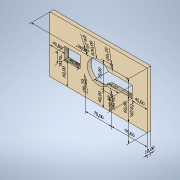
# Autodesk Inventor part: MotorHalterung
Saved by Autodesk Inventor 2020.3 (Build 243373010, 373A)
## iProperties
Created: 2021-02-04
Part Number: MotorHalterung
Material: Generisch
Document SubType Name: Modeling
Designer: Stefan
Density: 1 g/cm^3
Appearance: Vorgabe
Author: Stefan
Autodesk Inventor part; units mm, degrees
ref_plane "YZ Plane" through (0, 0, 0) normal (1, 0, 0) x (0, 1, 0)
ref_plane "XZ Plane" through (0, 0, 0) normal (0, 1, 0) x (-1, 0, 0)
ref_plane "XY Plane" through (0, 0, 0) normal (0, 0, 1) x (1, 0, 0)
sketch "Skizze2" plane through (0, 0, 0) normal (0, 0, 1) x (1, 0, 0)
  line L0 (145, 0) -> (260, 0)
  line L1 (260, 0) -> (260, 150)
  line L2 (260, 150) -> (0, 150)
  line L3 (0, 150) -> (0, 0)
  line L4 (0, 0) -> (145, 0)
  circle A0 centre (165.0018, 110.0018) radius 3.1
  circle A1 centre (165.0018, 39.9982) radius 3.1
  circle A2 centre (94.9982, 39.9982) radius 3.1
  circle A3 centre (94.9982, 110.0018) radius 3.1
  arc A4 (155.9808, 90) -> (155.9808, 60) centre (130, 75) ccw
  line L5 (155.9808, 90) -> (220, 90)
  line L6 (220, 90) -> (220, 60)
  line L7 (220, 60) -> (155.9808, 60)
  line L8 (40, 90) -> (80.5, 90)
  line L9 (80.5, 90) -> (80.5, 60)
  line L10 (80.5, 60) -> (40, 60)
  line L11 (40, 60) -> (40, 90)
  dimension "d13" = 6.2
  dimension "d14" = 30
  dimension "d15" = 90
  dimension "d16" = 90
  dimension "d17" = 90
  dimension "d18" = 40
  dimension "d19" = 179.5
  dimension "d20" = 220
  dimension "d21" = 260
  dimension "d22" = 150
  dimension "d23" = 60
  dimension "d24" = 90
  dimension "d25" = 260
  dimension "d26" = 0
  dimension "d27" = 90
  dimension "d28" = 60
  dimension "d29" = 150
  dimension "d30" = 150
  dimension "d31" = 0
  dimension "d32" = 0
  dimension "d33" = 150
  dimension "d34" = 0
  dimension "d35" = 0
  dimension "d36" = 0
  dimension "d37" = 0
  dimension "d38" = 90
  dimension "d39" = 40
  dimension "d40" = 40
  dimension "d41" = 90
  dimension "d42" = 60
  dimension "d43" = 40
  dimension "d44" = 40
  dimension "d45" = 60
  dimension "d46" = 94.9982
  dimension "d47" = 110.0018
  dimension "d48" = 94.9982
  dimension "d49" = 39.9982
  dimension "d50" = 104.0192
  dimension "d51" = 104.0192
  dimension "d52" = 115
  dimension "d53" = 115
  dimension "d54" = 115
  dimension "d55" = 0
  dimension "d56" = 165.0018
  dimension "d57" = 110.0018
  dimension "d58" = 165.0018
  dimension "d59" = 39.9982
  dimension "d60" = 90
  dimension "d61" = 179.5
  dimension "d62" = 179.5
  dimension "d63" = 90
  dimension "d64" = 60
  dimension "d65" = 179.5
  dimension "d66" = 179.5
  dimension "d67" = 30
  dimension "d68" = 90
  dimension "d69" = 220
  dimension "d70" = 220
  dimension "d71" = 90
  dimension "d72" = 60
  dimension "d73" = 220
  dimension "d74" = 220
  dimension "d75" = 60
  dimension "d76" = 150
  constraints: 24 end point, 7 parallel, 5 centre point, 3 equal radius, 2 point on circle, 1 horizontal, 1 vertical
  measures "d13" diameter of A0
  measures "d14" radius of A4
  measures "d15" angle of L1 L0
  measures "d16" angle of L1 L5
  measures "d17" angle of L1 L7
  measures "d18" distance between parallel lines of L1 L6
  measures "d19" distance between parallel lines of L1 L9
  measures "d20" distance between parallel lines of L1 L11
  measures "d21" distance between parallel lines of L1 L3
  measures "d22" distance between parallel lines of L2 L4
  measures "d23" distance between parallel lines of L2 L8
  measures "d24" distance between parallel lines of L2 L10
  measures "d25" distance from line of point (0, 0) L1
  measures "d26" distance from line of point (0, 0) L0
  measures "d27" distance from line of point (0, 0) L5
  measures "d28" distance from line of point (0, 0) L7
  measures "d29" distance from line of point (0, 0) L2
  measures "d30" distance from line of L1.end L0
  measures "d31" distance from line of L2.start L1
  measures "d32" distance from line of point (260, 150) L1
  measures "d33" distance from line of point (260, 150) L0
  measures "d34" distance from line of L0.end L1
  measures "d35" distance from line of L1.start L0
  measures "d36" distance from line of point (260, 0) L1
  measures "d37" distance from line of point (260, 0) L0
  measures "d38" distance from line of L6.start L0
  measures "d39" distance from line of L5.end L1
  measures "d40" distance from line of point (220, 90) L1
  measures "d41" distance from line of point (220, 90) L0
  measures "d42" distance from line of L6.end L0
  measures "d43" distance from line of L7.start L1
  measures "d44" distance from line of point (220, 60) L1
  measures "d45" distance from line of point (220, 60) L0
  measures "d46" distance from line of A0.centre L1
  measures "d47" distance from line of A0.centre L0
  measures "d48" distance from line of A1.centre L1
  measures "d49" distance from line of A1.centre L0
  measures "d50" distance from line of L5.start L1
  measures "d51" distance from line of L7.end L1
  measures "d52" distance from line of L0.start L1
  measures "d53" distance from line of L4.end L1
  measures "d54" distance from line of point (145, 0) L1
  measures "d55" distance from line of point (145, 0) L0
  measures "d56" distance from line of A3.centre L1
  measures "d57" distance from line of A3.centre L0
  measures "d58" distance from line of A2.centre L1
  measures "d59" distance from line of A2.centre L0
  measures "d60" distance from line of L9.start L0
  measures "d61" distance from line of L8.end L1
  measures "d62" distance from line of point (80.5, 90) L1
  measures "d63" distance from line of point (80.5, 90) L0
  measures "d64" distance from line of L9.end L0
  measures "d65" distance from line of L10.start L1
  measures "d66" distance from line of point (80.5, 60) L1
  measures "d67" distance from line of point (80.5, 60) L5
  measures "d68" distance from line of L11.end L0
  measures "d69" distance from line of L8.start L1
  measures "d70" distance from line of point (40, 90) L1
  measures "d71" distance from line of point (40, 90) L0
  measures "d72" distance from line of L11.start L0
  measures "d73" distance from line of L10.end L1
  measures "d74" distance from line of point (40, 60) L1
  measures "d75" distance from line of point (40, 60) L0
  measures "d76" distance from line of L3.start L0
extrude "Extrusion1" add sketch "Skizze2" along normal blind 10
